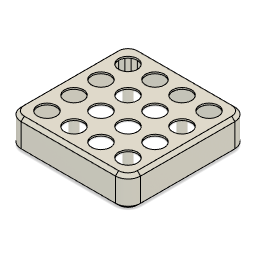
Case v13 (Autodesk Fusion 360 design; units mm, degrees)
Autodesk Fusion 360 part; units mm, degrees
note: some values were not read from the file. Set by a fixed rule: which sketch regions a step uses.
sketch "Length+Width" plane through (0, 0, 0) normal (0, 1, 0) x (1, 0, 0)
  line L0 (-76.2, -76.2) -> (76.2, -76.2)
  line L1 (76.2, -76.2) -> (76.2, 76.2)
  line L2 (76.2, 76.2) -> (-76.2, 76.2)
  line L3 (-76.2, 76.2) -> (-76.2, -76.2)
  line L4 (-76.2, -76.2) -> (76.2, 76.2) construction
  line L5 (76.2, -76.2) -> (-76.2, 76.2) construction
  dimension "d1" = 152.4
  dimension "d2" = 152.4
  constraint horizontal L0
  constraint perpendicular L0 L1
  constraint parallel L0 L2
  constraint parallel L1 L3
  constraint coincident L4 origin
  constraint coincident L5 origin
  measures "d1" distance of L1.end L2.end
  measures "d2" distance of L0.end L1.end
extrude "Extrude1" add sketch "Length+Width" along normal blind 38.1 makes body 1
fillet "Fillet1" radius 16 4 edges at (76.2, 19.05, 76.2) (-76.2, 19.05, 76.2) (-76.2, 19.05, -76.2) (76.2, 19.05, -76.2) on bodies 1
chamfer "Chamfer1" distance 4 angle 45 16 edges at (0, 38.1, -76.2) (-71.5137, 38.1, -71.5137) (-76.2, 38.1, 0) (-71.5137, 38.1, 71.5137) (0, 38.1, 76.2) (71.5137, 38.1, 71.5137) (76.2, 38.1, 0) (71.5137, 38.1, -71.5137) (0, 0, -76.2) (-71.5137, 0, -71.5137) (-76.2, 0, 0) (-71.5137, 0, 71.5137) (0, 0, 76.2) (71.5137, 0, 71.5137) (76.2, 0, 0) (71.5137, 0, -71.5137) on bodies 1
sketch "Button Holes" plane through (0, 38.1, 0) normal (0, 1, 0) x (-1, 0, 0)
  line L0 (-60.2, -72.2) -> (60.2, -72.2)
  arc A0 (60.2, -72.2) -> (72.2, -60.2) centre (60.2, -60.2) ccw
  line L1 (72.2, -60.2) -> (72.2, 60.2)
  arc A1 (72.2, 60.2) -> (60.2, 72.2) centre (60.2, 60.2) ccw
  line L2 (60.2, 72.2) -> (-60.2, 72.2)
  arc A2 (-60.2, 72.2) -> (-72.2, 60.2) centre (-60.2, 60.2) ccw
  line L3 (-72.2, 60.2) -> (-72.2, -60.2)
  arc A3 (-72.2, -60.2) -> (-60.2, -72.2) centre (-60.2, -60.2) ccw
  line L4 (60.2, 60.2) -> (-60.2, 60.2) construction
  line L5 (-60.2, 60.2) -> (-60.2, -60.2) construction
  line L6 (-60.2, -60.2) -> (60.2, -60.2) construction
  line L7 (60.2, -60.2) -> (60.2, 60.2) construction
  line L8 (60.2, 60.2) -> (-60.2, -60.2) construction
  circle A4 centre (51.7147, 51.7147) radius 12
  circle A5 centre (51.7147, 51.7147) radius 13.6
  line L9 (68.6853, -68.6853) -> (-68.6853, 68.6853) construction
  circle A6 centre (-51.7147, -51.7147) radius 12
  circle A7 centre (-51.7147, -51.7147) radius 13.6
  line L10 (51.7147, 51.7147) -> (-51.7147, 51.7147) construction
  line L11 (-51.7147, 51.7147) -> (-51.7147, -51.7147) construction
  line L12 (-51.7147, -51.7147) -> (51.7147, -51.7147) construction
  line L13 (51.7147, -51.7147) -> (51.7147, 51.7147) construction
  circle A8 centre (17.2382, 51.7147) radius 13.6
  circle A9 centre (17.2382, 51.7147) radius 12
  circle A10 centre (-17.2382, 51.7147) radius 13.6
  circle A11 centre (-17.2382, 51.7147) radius 12
  circle A12 centre (-51.7147, 51.7147) radius 13.6
  circle A13 centre (-51.7147, 51.7147) radius 12
  circle A14 centre (51.7147, 17.2382) radius 13.6
  circle A15 centre (51.7147, 17.2382) radius 12
  circle A16 centre (17.2382, 17.2382) radius 13.6
  circle A17 centre (17.2382, 17.2382) radius 12
  circle A18 centre (-17.2382, 17.2382) radius 13.6
  circle A19 centre (-17.2382, 17.2382) radius 12
  circle A20 centre (-51.7147, 17.2382) radius 13.6
  circle A21 centre (-51.7147, 17.2382) radius 12
  circle A22 centre (51.7147, -17.2382) radius 13.6
  circle A23 centre (51.7147, -17.2382) radius 12
  circle A24 centre (17.2382, -17.2382) radius 13.6
  circle A25 centre (17.2382, -17.2382) radius 12
  circle A26 centre (-17.2382, -17.2382) radius 13.6
  circle A27 centre (-17.2382, -17.2382) radius 12
  circle A28 centre (-51.7147, -17.2382) radius 13.6
  circle A29 centre (-51.7147, -17.2382) radius 12
  circle A30 centre (51.7147, -51.7147) radius 13.6
  circle A31 centre (51.7147, -51.7147) radius 12
  circle A32 centre (17.2382, -51.7147) radius 13.6
  circle A33 centre (17.2382, -51.7147) radius 12
  circle A34 centre (-17.2382, -51.7147) radius 13.6
  circle A35 centre (-17.2382, -51.7147) radius 12
  circle A36 centre (-51.7147, -51.7147) radius 13.6
  circle A37 centre (-51.7147, -51.7147) radius 12
  dimension "d8" = 24
  dimension "d9" = 27.2
  dimension "d11" = 103.4294
  dimension "d14" = -103.4294
  dimension "d15" = -103.4294
  constraint horizontal L4
  constraint vertical L5
  constraint horizontal L6
  constraint vertical L7
  constraint coincident A3.centre L5.end
  constraint coincident A1.centre L4.start
  constraint coincident A1.centre A4
  constraint concentric A4 A5
  constraint midpoint A0 L9.start
  constraint midpoint A2 L9.end
  constraint symmetric A4 L9 A6
  constraint symmetric A5 L9 A7
  constraint horizontal L10
  constraint vertical L11
  constraint horizontal L12
  constraint vertical L13
  constraint coincident A6.centre A7.centre
  constraint coincident A4.centre A5.centre
  measures "d8" diameter of A4
  measures "d9" diameter of A5
  measures "d11" distance of A4.centre L12.end
sketch "Bottom Splitting Tool" plane through (-76.2, 0, 0) normal (-1, 0, 0) x (0, 0, 1)
  line L0 (-60.2, 4) -> (60.2, 4)
  line L1 (60.2, 4) -> (60.2, 34.1)
  line L2 (60.2, 34.1) -> (-60.2, 34.1)
  line L3 (-60.2, 34.1) -> (-60.2, 4)
  line L4 (-60.2, 4) -> (60.2, 4)
  constraint coincident L0.start L3.end
  constraint coincident L0.end L1.start
split "Split1" by curves path "Bottom Splitting Tool" along L4 bodies 1 makes body 2 at (20.0667, 0, -24.0667)
combine "Combine1" operation add target body 2 tool bodies 1
extrude "Extrude2" cut 1 faces at (20.0667, 0, -24.0667) along direction (0, 1, 0) blind 36.1 on bodies 2 bodies 2
extrude "Extrude3" cut sketch "Button Holes" against normal blind 2 contours A4 | A6 A37 | A9 | A11 | A13 | A15 | A17 | A19 | A21 | A23 | A25 | A27 | A29 | A31 | A33 | A35 bodies 2
sketch "Inside M4 Nut Inserts+Screw Posts" plane through (0, 36.1, 0) normal (0, -1, 0) x (1, 0, 0)
  circle A0 centre (51.7147, 17.2382) radius 12
  circle A1 centre (17.2382, -17.2382) radius 12
  circle A2 centre (-17.2382, 17.2382) radius 12
  circle A3 centre (-51.7147, -17.2382) radius 12
  circle A4 centre (-51.7147, 17.2382) radius 12
  circle A5 centre (-17.2382, -17.2382) radius 12
  circle A6 centre (17.2382, 17.2382) radius 12
  circle A7 centre (51.7147, -17.2382) radius 12
  circle A8 centre (51.7147, 51.7147) radius 12
  circle A9 centre (17.2382, -51.7147) radius 12
  circle A10 centre (-17.2382, 51.7147) radius 12
  circle A11 centre (-51.7147, -51.7147) radius 12
  circle A12 centre (-51.7147, 51.7147) radius 12
  circle A13 centre (-17.2382, -51.7147) radius 12
  circle A14 centre (17.2382, 51.7147) radius 12
  circle A15 centre (51.7147, -51.7147) radius 12
  line L0 (-60.2, -72.2) -> (60.2, -72.2)
  arc A16 (60.2, -72.2) -> (72.2, -60.2) centre (60.2, -60.2) ccw
  line L1 (72.2, -60.2) -> (72.2, 60.2)
  arc A17 (72.2, 60.2) -> (60.2, 72.2) centre (60.2, 60.2) ccw
  line L2 (60.2, 72.2) -> (-60.2, 72.2)
  arc A18 (-60.2, 72.2) -> (-72.2, 60.2) centre (-60.2, 60.2) ccw
  line L3 (-72.2, 60.2) -> (-72.2, -60.2)
  arc A19 (-72.2, -60.2) -> (-60.2, -72.2) centre (-60.2, -60.2) ccw
  line L4 (60.2, 72.2) -> (60.2, 60.2)
  line L5 (72.2, 60.2) -> (60.2, 60.2)
  line L6 (60.2, -72.2) -> (60.2, -60.2)
  line L7 (60.2, -60.2) -> (72.2, -60.2)
  line L8 (0, -72.2) -> (0, 72.2) construction
  line L9 (-60.2, 72.2) -> (-60.2, 60.2)
  line L10 (-72.2, 60.2) -> (-60.2, 60.2)
  arc A20 (-60.2, 72.2) -> (-72.2, 60.2) centre (-60.2, 60.2) ccw
  line L11 (-60.2, -60.2) -> (-72.2, -60.2)
  line L12 (-60.2, -72.2) -> (-60.2, -60.2)
  arc A21 (-72.2, -60.2) -> (-60.2, -72.2) centre (-60.2, -60.2) ccw
  line L13 (-72.2, 0) -> (72.2, 0) construction
  line L14 (-51.7147, -17.2382) -> (-17.2382, -17.2382) construction
  line L15 (-17.2382, -17.2382) -> (-17.2382, -51.7147) construction
  line L16 (-17.2382, -51.7147) -> (-51.7147, -51.7147) construction
  line L17 (-51.7147, -51.7147) -> (-51.7147, -17.2382) construction
  line L18 (-51.7147, -17.2382) -> (-17.2382, -51.7147) construction
  line L19 (-51.7147, -51.7147) -> (-17.2382, -17.2382) construction
  circle A22 centre (-34.4765, -34.4765) radius 5
  line L20 (-34.4765, -29.4765) -> (-34.4765, -39.4765)
  line L21 (-34.4765, -38.3065) -> (-31.1596, -36.3915)
  line L22 (-31.1596, -36.3915) -> (-31.1596, -32.5615)
  line L23 (-31.1596, -32.5615) -> (-34.4765, -30.6465)
  line L24 (-34.4765, -30.6465) -> (-37.7934, -32.5615)
  line L25 (-37.7934, -32.5615) -> (-37.7934, -36.3915)
  line L26 (-37.7934, -36.3915) -> (-34.4765, -38.3065)
  circle A23 centre (-34.4765, -34.4765) radius 2
  circle A24 centre (34.4765, -34.4765) radius 2
  line L27 (31.1596, -36.3915) -> (31.1596, -32.5615)
  line L28 (31.1596, -32.5615) -> (34.4765, -30.6465)
  line L29 (34.4765, -30.6465) -> (37.7934, -32.5615)
  line L30 (37.7934, -32.5615) -> (37.7934, -36.3915)
  line L31 (37.7934, -36.3915) -> (34.4765, -38.3065)
  line L32 (34.4765, -38.3065) -> (31.1596, -36.3915)
  circle A25 centre (34.4765, -34.4765) radius 5
  circle A26 centre (34.4765, 34.4765) radius 2
  line L33 (37.7934, 36.3915) -> (34.4765, 38.3065)
  line L34 (34.4765, 38.3065) -> (31.1596, 36.3915)
  line L35 (31.1596, 36.3915) -> (31.1596, 32.5615)
  line L36 (31.1596, 32.5615) -> (34.4765, 30.6465)
  line L37 (34.4765, 30.6465) -> (37.7934, 32.5615)
  line L38 (37.7934, 32.5615) -> (37.7934, 36.3915)
  circle A27 centre (34.4765, 34.4765) radius 5
  circle A28 centre (-34.4765, 34.4765) radius 2
  line L39 (-31.1596, 36.3915) -> (-31.1596, 32.5615)
  line L40 (-31.1596, 32.5615) -> (-34.4765, 30.6465)
  line L41 (-34.4765, 30.6465) -> (-37.7934, 32.5615)
  line L42 (-37.7934, 32.5615) -> (-37.7934, 36.3915)
  line L43 (-34.4765, 38.3065) -> (-31.1596, 36.3915)
  circle A29 centre (-34.4765, 34.4765) radius 5
  line L44 (-37.7934, 36.3915) -> (-34.4765, 38.3065)
  point P0 (-34.4765, -34.4765)
  dimension "d35" = 10
  dimension "d36" = 3.83
  dimension "d37" = 4
  constraint coincident A17.end L2.start
  constraint coincident A17.centre L4.end
  constraint coincident L1.end A17.start
  constraint coincident L0.end A16.start
  constraint coincident A16.centre L6.end
  constraint coincident A16.end L1.start
  constraint midpoint L0 L8.start
  constraint midpoint L2 L8.end
  constraint symmetric L0.end L8 L0.start
  constraint symmetric A16.end L8 L3.end
  constraint symmetric A16 L8 A21
  constraint symmetric L1.end L8 A18.end
  constraint symmetric A17.end L8 L2.end
  constraint symmetric A17 L8 A20
  constraint symmetric A17.centre L8 A18.centre
  constraint symmetric A16.centre L8 A19.centre
  constraint midpoint L3 L13.start
  constraint midpoint L1 L13.end
  constraint horizontal L14
  constraint vertical L15
  constraint horizontal L16
  constraint vertical L17
  constraint coincident A13.centre L15.end
  constraint coincident A3.centre L14.start
  constraint coincident A5.centre L14.end
  constraint midpoint L18 P0
  constraint coincident A22 L20.start
  constraint coincident A22 L20.end
  constraint vertical L20
  constraint coincident P0 A22.centre
  constraint concentric A22 A23
  constraint symmetric L8 A22 A25
  constraint symmetric L8 L21.start L31.end
  constraint symmetric L8 L21.end L27.start
  constraint symmetric L8 L22.end L27.end
  constraint symmetric L8 L23.end L28.end
  constraint symmetric L8 L24.end L29.end
  constraint symmetric L8 L25.end L30.end
  constraint symmetric L8 A23 A24
  constraint symmetric L13 A22 A29
  constraint symmetric L13 L21.start L43.start
  constraint symmetric L13 L21.end L39.start
  constraint symmetric L13 L22.end L39.end
  constraint symmetric L13 L23.end L40.end
  constraint symmetric L13 L24.end L41.end
  constraint symmetric L13 L25.end L42.end
  constraint symmetric L13 A23 A28
  constraint symmetric L13 A24 A26
  constraint symmetric L13 L27.start L34.end
  constraint symmetric L13 L27.end L35.end
  constraint symmetric L13 L28.end L36.end
  constraint symmetric L13 L29.end L37.end
  constraint symmetric L13 L30.end L33.start
  constraint symmetric L13 L31.end L33.end
  constraint symmetric L13 A25 A27
  measures "d35" diameter of A22
  measures "d36" distance of L21.start P0
  measures "d37" diameter of A23
extrude "Extrude4" add sketch "Inside M4 Nut Inserts+Screw Posts" along normal blind 34.1 contours A17 L4 L5 | A18 L9 L10 A20 | A16 L6 L7 | A19 L11 L12 A21 bodies 2
fillet "Fillet2" radius 4 2 edges at (-60.2, 19.05, 60.2) (60.2, 19.05, 60.2) on bodies 2
fillet "Fillet2" radius 4 2 edges at (-60.2, 19.05, -60.2) (60.2, 19.05, -60.2) on bodies 2
sketch "Outside M4 Nut Inserts" plane through (0, 2, 0) normal (0, -1, 0) x (1, 0, 0)
  arc A0 (-60.2, -64.2) -> (-64.2, -60.2) centre (-64.2, -64.2) ccw
  line L0 (-64.2, -60.2) -> (-72.2, -60.2)
  arc A1 (-72.2, -60.2) -> (-60.2, -72.2) centre (-60.2, -60.2) ccw
  line L1 (-60.2, -72.2) -> (-60.2, -64.2)
  line L2 (-68.6853, -68.6853) -> (-61.3716, -61.3716) construction
  line L3 (-65.0284, -68.8584) -> (-61.7115, -66.9434)
  line L4 (-61.7115, -66.9434) -> (-61.7115, -63.1134)
  line L5 (-61.7115, -63.1134) -> (-65.0284, -61.1984)
  line L6 (-65.0284, -61.1984) -> (-68.3453, -63.1134)
  line L7 (-68.3453, -63.1134) -> (-68.3453, -66.9434)
  line L8 (-68.3453, -66.9434) -> (-65.0284, -68.8584)
  line L9 (0, 70) -> (0, -70) construction
  line L10 (-70, 0) -> (70, 0) construction
  line L11 (65.0284, -61.1984) -> (68.3453, -63.1134)
  line L12 (68.3453, -63.1134) -> (68.3453, -66.9434)
  line L13 (68.3453, -66.9434) -> (65.0284, -68.8584)
  line L14 (65.0284, -68.8584) -> (61.7115, -66.9434)
  line L15 (61.7115, -66.9434) -> (61.7115, -63.1134)
  line L16 (61.7115, -63.1134) -> (65.0284, -61.1984)
  line L17 (-65.0284, 61.1984) -> (-68.3453, 63.1134)
  line L18 (-68.3453, 63.1134) -> (-68.3453, 66.9434)
  line L19 (-68.3453, 66.9434) -> (-65.0284, 68.8584)
  line L20 (-65.0284, 68.8584) -> (-61.7115, 66.9434)
  line L21 (-61.7115, 66.9434) -> (-61.7115, 63.1134)
  line L22 (-61.7115, 63.1134) -> (-65.0284, 61.1984)
  line L23 (61.7115, 66.9434) -> (61.7115, 63.1134)
  line L24 (65.0284, 68.8584) -> (61.7115, 66.9434)
  line L25 (68.3453, 66.9434) -> (65.0284, 68.8584)
  line L26 (68.3453, 63.1134) -> (68.3453, 66.9434)
  line L27 (65.0284, 61.1984) -> (68.3453, 63.1134)
  line L28 (61.7115, 63.1134) -> (65.0284, 61.1984)
  circle A2 centre (-65.0284, -65.0284) radius 2
  circle A3 centre (65.0284, -65.0284) radius 2
  circle A4 centre (-65.0284, 65.0284) radius 2
  circle A5 centre (65.0284, 65.0284) radius 2
  point P0 (-65.0284, -65.0284)
  point P1 (65.0284, 65.0284)
  point P2 (-65.0284, 65.0284)
  dimension "d29" = 3.83
  dimension "d32" = 4
  constraint midpoint A1 L2.start
  constraint midpoint A0 L2.end
  constraint midpoint L2 P0
  constraint vertical L9
  constraint horizontal L10
  constraint symmetric L3.start L9 L13.end
  constraint symmetric L3.end L9 L14.end
  constraint symmetric L4.end L9 L15.end
  constraint symmetric L5.end L9 L11.start
  constraint symmetric L6.end L9 L11.end
  constraint symmetric L7.end L9 L12.end
  constraint symmetric L3.start L10 L19.end
  constraint symmetric L3.end L10 L20.end
  constraint symmetric L4.end L10 L21.end
  constraint symmetric L5.end L10 L17.start
  constraint symmetric L6.end L10 L17.end
  constraint symmetric L7.end L10 L18.end
  constraint symmetric L10 L11.start L27.start
  constraint symmetric L10 L11.end L26.start
  constraint symmetric L10 L12.end L25.start
  constraint symmetric L10 L13.end L24.start
  constraint symmetric L10 L14.end L23.start
  constraint symmetric L10 L15.end L23.end
  constraint coincident P0 A2.centre
  constraint symmetric L9 A2 A3
  constraint symmetric L10 P0 P2
  constraint symmetric L10 A3.centre P1
  constraint symmetric L10 A2 A4
  constraint symmetric L10 A3 A5
  measures "d29" distance of L3.start P0
  measures "d32" diameter of A2
extrude "Extrude5" cut sketch "Outside M4 Nut Inserts" against normal blind 3.2 contours L3 L4 L5 L6 L7 L8 | L11 L12 L13 L14 L15 L16 | L17 L18 L19 L20 L21 L22 | L23 L24 L25 L26 L27 L28 | A2 | A3 | A4 | A5 bodies 2
extrude "Extrude6" cut sketch "Outside M4 Nut Inserts" against normal blind 4.2 contours A2 | A3 | A4 | A5 bodies 2
extrude "Extrude7" add sketch "Inside M4 Nut Inserts+Screw Posts" along normal blind 30 contours A22 L20 L21 L22 L23 | A22 L20 L24 L25 L26 | A25 | A27 | A29 bodies 2
extrude "Extrude8" add sketch "Inside M4 Nut Inserts+Screw Posts" along normal blind 26.8 contours L20 L21 L22 L23 A23 | L20 L24 L25 L26 A23 | L27 L28 L29 L30 L31 L32 | L33 L34 L35 L36 L37 L38 | L39 L40 L41 L42 L43 L44 bodies 2
extrude "Extrude9" add sketch "Inside M4 Nut Inserts+Screw Posts" along normal blind 25.8 contours L20 A23 | L20 A23 | A24 | A26 | A28 bodies 2
sketch "Bottom Cover Footprint" plane through (0, 36.1, 0) normal (0, -1, 0) x (1, 0, 0)
  circle A0 centre (34.4765, 34.4765) radius 5
  circle A1 centre (-34.4765, 34.4765) radius 5
  line L0 (64.2, -60.2) -> (72.2, -60.2)
  line L1 (72.2, -60.2) -> (72.2, 60.2)
  line L2 (72.2, 60.2) -> (64.2, 60.2)
  arc A2 (60.2, 64.2) -> (64.2, 60.2) centre (64.2, 64.2) ccw
  line L3 (60.2, 64.2) -> (60.2, 72.2)
  line L4 (60.2, 72.2) -> (-60.2, 72.2)
  line L5 (-60.2, 72.2) -> (-60.2, 64.2)
  arc A3 (-64.2, 60.2) -> (-60.2, 64.2) centre (-64.2, 64.2) ccw
  line L6 (-64.2, 60.2) -> (-72.2, 60.2)
  line L7 (-72.2, 60.2) -> (-72.2, -60.2)
  line L8 (-72.2, -60.2) -> (-64.2, -60.2)
  arc A4 (-60.2, -64.2) -> (-64.2, -60.2) centre (-64.2, -64.2) ccw
  line L9 (-60.2, -64.2) -> (-60.2, -72.2)
  line L10 (-60.2, -72.2) -> (60.2, -72.2)
  line L11 (60.2, -72.2) -> (60.2, -64.2)
  arc A5 (64.2, -60.2) -> (60.2, -64.2) centre (64.2, -64.2) ccw
  circle A6 centre (51.7147, -51.7147) radius 12
  circle A7 centre (-51.7147, -51.7147) radius 12
  circle A8 centre (51.7147, 51.7147) radius 12
  circle A9 centre (-51.7147, 51.7147) radius 12
  circle A10 centre (17.2382, 51.7147) radius 12
  circle A11 centre (-17.2382, -51.7147) radius 12
  circle A12 centre (-17.2382, 51.7147) radius 12
  circle A13 centre (17.2382, -51.7147) radius 12
  circle A14 centre (51.7147, -17.2382) radius 12
  circle A15 centre (17.2382, 17.2382) radius 12
  circle A16 centre (-17.2382, -17.2382) radius 12
  circle A17 centre (-51.7147, 17.2382) radius 12
  circle A18 centre (-51.7147, -17.2382) radius 12
  circle A19 centre (-17.2382, 17.2382) radius 12
  circle A20 centre (17.2382, -17.2382) radius 12
  circle A21 centre (51.7147, 17.2382) radius 12
  circle A22 centre (-34.4765, -34.4765) radius 5
  circle A23 centre (34.4765, -34.4765) radius 5
  arc A24 (-60.2, 72.2) -> (-72.2, 60.2) centre (-60.2, 60.2) ccw
  arc A25 (-72.2, -60.2) -> (-60.2, -72.2) centre (-60.2, -60.2) ccw
  arc A26 (60.2, -72.2) -> (72.2, -60.2) centre (60.2, -60.2) ccw
  arc A27 (72.2, 60.2) -> (60.2, 72.2) centre (60.2, 60.2) ccw
  line L12 (-60.2, 72.2) -> (60.2, 72.2)
  line L13 (72.2, 60.2) -> (72.2, -60.2)
  line L14 (60.2, -72.2) -> (-60.2, -72.2)
  line L15 (-72.2, -60.2) -> (-72.2, 60.2)
  constraint tangent L7 A24
  constraint coincident L6.end L7.start
  constraint coincident L4.end L5.start
  constraint tangent L10 A25
  constraint tangent L7 A25
  constraint coincident L9.end L10.start
  constraint tangent L1 A26
  constraint coincident L0.end L1.start
  constraint coincident L10.end L11.start
  constraint tangent L1 A27
  constraint coincident L1.end L2.start
  constraint coincident L3.end L4.start
  constraint tangent A24 L15
equation "d1 = 6\""
equation "d2 = d1"
equation "d14 = -d11"
equation "d15 = -d11"
equation "d29 = ( 7.66 / 2 ) * 1 mm"
equation "d36 = ( 7.66 / 2 ) * 1 mm"
equation "d40 = 30 mm - 3.2 mm"
equation "d42 = ( 30 mm - 3.2 mm ) - 1 mm"
named bodies: "Case"
